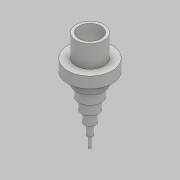
# Autodesk Inventor part: exercise1-3
Saved by Autodesk Inventor 2018 (Build 220112000, 112)
## iProperties
Created: 2020-09-19
Part Number: exercise1-3
Material: 一般
Document SubType Name: Modeling
Designer: 王鼎鈞
Density: 1 g/cm^3
Appearance: 預設
Author: 王鼎鈞
Autodesk Inventor part; units mm, degrees
ref_plane "YZ Plane" through (0, 0, 0) normal (1, 0, 0) x (0, 1, 0)
ref_plane "XZ Plane" through (0, 0, 0) normal (0, 1, 0) x (-1, 0, 0)
ref_plane "XY Plane" through (0, 0, 0) normal (0, 0, 1) x (1, 0, 0)
sketch "草圖1" plane through (0, 0, 0) normal (1, 0, 0) x (0, 1, 0)
  line L0 (-8, 0) -> (48, 0) projected
  line L1 (0, -156) -> (0, 96) projected
  line L2 (0, 0) -> (40, 0)
  line L3 (40, 0) -> (40, 20)
  line L4 (40, 20) -> (0, 20)
  line L5 (0, 20) -> (0, 0)
  line L6 (0, 20) -> (25, 20)
  line L7 (25, 20) -> (25, 60)
  line L8 (25, 60) -> (0, 60)
  line L9 (0, 60) -> (0, 20)
  line L10 (0, 20) -> (20, 20)
  line L11 (20, 20) -> (20, 60)
  line L12 (20, 60) -> (0, 60)
  line L13 (0, 60) -> (0, 20)
  line L14 (0, 0) -> (25, 0)
  line L15 (25, 0) -> (25, -20)
  line L16 (25, -20) -> (0, -20)
  line L17 (0, -20) -> (0, 0)
  line L18 (0, -20) -> (20, -20)
  line L19 (20, -20) -> (20, -40)
  line L20 (20, -40) -> (0, -40)
  line L21 (0, -40) -> (0, -20)
  line L22 (0, -40) -> (15, -40)
  line L23 (15, -40) -> (15, -60)
  line L24 (15, -60) -> (0, -60)
  line L25 (0, -60) -> (0, -40)
  line L26 (0, -60) -> (10, -60)
  line L27 (10, -60) -> (10, -80)
  line L28 (10, -80) -> (0, -80)
  line L29 (0, -80) -> (0, -60)
  line L30 (0, -80) -> (5, -80)
  line L31 (5, -80) -> (5, -100)
  line L32 (5, -100) -> (0, -100)
  line L33 (0, -100) -> (0, -80)
  line L34 (0, -100) -> (2.5, -100)
  line L35 (2.5, -100) -> (2.5, -120)
  line L36 (2.5, -120) -> (0, -120)
  line L37 (0, -120) -> (0, -100)
  dimension "d0" = 40
  dimension "d1" = 20
  dimension "d2" = 25
  dimension "d3" = 40
  dimension "d4" = 20
  dimension "d5" = 25
  dimension "d6" = 20
  dimension "d7" = 20
  dimension "d8" = 20
  dimension "d9" = 15
  dimension "d10" = 20
  dimension "d11" = 10
  dimension "d12" = 20
  dimension "d13" = 5
  dimension "d14" = 20
  dimension "d15" = 2.5
  dimension "d16" = 20
  constraints: 72 end point, 18 parallel, 9 horizontal, 9 perpendicular, 1 point on line
  measures "d0" distance of L4.end L3.end
  measures "d1" distance of L3.end L2.end
  measures "d2" distance of L8.end L7.end
  measures "d3" distance of L7.end L6.end
  measures "d4" distance of L12.end L11.end
  measures "d5" distance of L15.end L16.end
  measures "d6" distance of L14.end L15.end
  measures "d7" distance of L19.end L20.end
  measures "d8" distance of L18.end L19.end
  measures "d9" distance of L23.end L24.end
  measures "d10" distance of L22.end L23.end
  measures "d11" distance of L27.end L28.end
  measures "d12" distance of L26.end L27.end
  measures "d13" distance of L31.end L32.end
  measures "d14" distance of L30.end L31.end
  measures "d15" distance of L35.end L36.end
  measures "d16" distance of L34.end L35.end
revolve "迴轉1" add sketch "草圖1" angle 360 about axis through (0, 0, -60) along (0, 0, 1) contours L1 L4 L3 L0 | L0 L15 L16 L1 | L16 L19 L20 L1 | L20 L23 L24 L1 | L11 L8 L7 L4 | L24 L27 L28 L1 | L28 L31 L32 L1 | L32 L35 L36 L1
